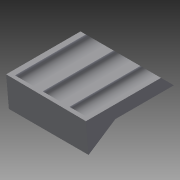
# Autodesk Inventor part: coin_holder_large_only
Saved by Autodesk Inventor 2015 (Build 190159000, 159)
## iProperties
Created: 2015-02-10
Part Number: coin_holder_large_only
Material: Generic
Document SubType Name: Modeling
Designer: Justin
Density: 1 g/cm^3
Appearance: Default
Author: Justin
Autodesk Inventor part; units mm, degrees
ref_plane "YZ Plane" through (0, 0, 0) normal (1, 0, 0) x (0, 1, 0)
ref_plane "XZ Plane" through (0, 0, 0) normal (0, 1, 0) x (-1, 0, 0)
sketch "Sketch1" plane through (0, 0, 0) normal (0, 0, 1) x (1, 0, 0)
  arc A0 (12.7973, -6.8176) -> (-12.597, -7.1809) centre (0, 0) ccw
  arc A1 (50.4829, -6.2785) -> (26.2017, -6.6259) centre (38.25, 0) ccw
  arc A2 (85.5853, -5.7763) -> (63.5844, -6.091) centre (74.5, 0) ccw
  arc A3 (117.8988, -5.314) -> (98.5072, -5.5914) centre (108.125, 0) ccw
  arc A4 (147.9764, -4.8837) -> (130.6669, -5.1313) centre (139.25, 0) ccw
  arc A5 (177.1345, -4.4665) -> (160.4967, -4.7045) centre (168.75, 0) ccw
  line L0 (-20, 20) -> (188.75, 20)
  line L1 (188.75, 20) -> (188.75, -4.3003)
  line L2 (-20, 20) -> (-20, -7.2868)
  line L3 (-20, -7.2868) -> (188.75, -4.3003)
  dimension "d0" = 29
  dimension "d1" = 27.5
  dimension "d2" = 25
  dimension "d3" = 22.25
  dimension "d4" = 20
  dimension "d5" = 19
  dimension "d6" = 38.25
  dimension "d7" = 36.25
  dimension "d8" = 33.625
  dimension "d9" = 31.125
  dimension "d10" = 29.5
  dimension "d11" = 0
  dimension "d12" = 0
  dimension "d13" = 0
  dimension "d14" = 0
  dimension "d15" = 0
  dimension "d20" = 20
  dimension "d22" = 20
  dimension "d23" = 20
  dimension "d24" = 7
  dimension "d25" = 4.586
  constraints: 12 point on circle, 6 centre point, 6 end point, 1 coincident, 1 horizontal, 1 perpendicular, 1 vertical, 15 other
  measures "d0" diameter of A0
  measures "d1" diameter of A1
  measures "d2" diameter of A2
  measures "d3" diameter of A3
  measures "d4" diameter of A4
  measures "d5" diameter of A5
  measures "d6" distance of A1.centre A0.centre
  measures "d7" distance of A2.centre A1.centre
  measures "d8" distance of A3.centre A2.centre
  measures "d9" distance of A4.centre A3.centre
  measures "d10" distance of A5.centre A4.centre
  measures "d11" vertical distance of point (0, 0) A1.centre
  measures "d12" vertical distance of A1.centre A2.centre
  measures "d13" vertical distance of A2.centre A3.centre
  measures "d14" vertical distance of A3.centre A4.centre
  measures "d15" vertical distance of A4.centre A5.centre
  measures "d20" distance from line of L0 A0.centre
  measures "d22" horizontal distance of A5.centre L0.end
  measures "d23" distance from line of L2 A0.centre
sketch "Sketch4" plane through (0, 0, 0) normal (1, 0, 0) x (0, 1, 0)
  line L0 (0, 0) -> (29.9033, -29.9033)
  line L1 (0, 5.9807) -> (0, -35.884) projected
  point P0 (100, 0)
  dimension "d51" = 45
  dimension "d53" = 0
  dimension "d55" = 29.9033
  dimension "d98" = 100
  constraints: 2 end point
  measures "d51" angle of L0 L1
  measures "d53" vertical distance of L0.start point (100, 0)
  measures "d55" horizontal distance of L0.start L0.end
  measures "d98" distance of L0.start point (100, 0)
ref_plane "Work Plane4" through (0, 100, 0) normal (0, 0.7071068, 0.7071068) x (1, 0, 0)
ref_plane "Work Plane3" through (-10, 0, 0) normal (0, 0.7071068, 0.7071068) x (1, 0, 0)
sketch "Sketch5" plane through (-10, 0, 0) normal (0, 0.7071068, 0.7071068) x (1, 0, 0)
  arc A0 (42.7973, 0.4692) -> (17.403, 0.1059) centre (30, 7.2868) ccw
  arc A1 (80.4829, 1.0084) -> (56.2017, 0.661) centre (68.25, 7.2868) ccw
  arc A2 (115.5853, 1.5106) -> (93.5844, 1.1958) centre (104.5, 7.2868) ccw
  arc A3 (147.8988, 1.9729) -> (128.5072, 1.6954) centre (138.125, 7.2868) ccw
  arc A4 (177.9764, 2.4032) -> (160.6669, 2.1555) centre (169.25, 7.2868) ccw
  arc A5 (207.1345, 2.8203) -> (190.4967, 2.5823) centre (198.75, 7.2868) ccw
  line L0 (10, 27.2868) -> (218.75, 27.2868)
  line L1 (218.75, 27.2868) -> (218.75, 2.9865)
  line L2 (10, 27.2868) -> (10, 0)
  line L3 (10, 0) -> (17.403, 0.1059)
  line L4 (42.7973, 0.4692) -> (56.2017, 0.661)
  line L5 (80.4829, 1.0084) -> (93.5844, 1.1958)
  line L6 (115.5853, 1.5106) -> (128.5072, 1.6954)
  line L7 (207.1345, 2.8203) -> (218.75, 2.9865)
  line L8 (147.8988, 1.9729) -> (160.6669, 2.1555)
  line L9 (177.9764, 2.4032) -> (190.4967, 2.5823)
  dimension "d56" = 29
  dimension "d57" = 27.5
  dimension "d58" = 25
  dimension "d59" = 22.25
  dimension "d60" = 20
  dimension "d61" = 19
  dimension "d62" = 38.25
  dimension "d63" = 36.25
  dimension "d64" = 33.625
  dimension "d65" = 31.125
  dimension "d66" = 29.5
  dimension "d67" = 0
  dimension "d68" = 0
  dimension "d69" = 0
  dimension "d70" = 0
  dimension "d71" = 0
  dimension "d72" = 20
  dimension "d73" = 20
  dimension "d74" = 20
  constraints: 20 end point, 12 point on circle, 6 centre point, 2 coincident, 1 horizontal, 1 perpendicular, 1 vertical
  measures "d56" diameter of A0
  measures "d57" diameter of A1
  measures "d58" diameter of A2
  measures "d59" diameter of A3
  measures "d60" diameter of A4
  measures "d61" diameter of A5
  measures "d62" distance of A1.centre A0.centre
  measures "d63" distance of A2.centre A1.centre
  measures "d64" distance of A3.centre A2.centre
  measures "d65" distance of A4.centre A3.centre
  measures "d66" distance of A5.centre A4.centre
  measures "d67" vertical distance of point (30, 7.287) A1.centre
  measures "d68" vertical distance of A1.centre A2.centre
  measures "d69" vertical distance of A2.centre A3.centre
  measures "d70" vertical distance of A3.centre A4.centre
  measures "d71" vertical distance of A4.centre A5.centre
  measures "d72" distance from line of L0 A0.centre
  measures "d73" horizontal distance of A5.centre L0.end
  measures "d74" distance from line of L2 A0.centre
sketch "Sketch6" plane through (0, 100, 0) normal (0, 0.7071068, 0.7071068) x (1, 0, 0)
  arc A0 (32.7973, 0.4692) -> (7.403, 0.1059) centre (20, 7.2868) ccw
  arc A1 (70.4829, 1.0084) -> (46.2017, 0.661) centre (58.25, 7.2868) ccw
  arc A2 (105.5853, 1.5106) -> (83.5844, 1.1958) centre (94.5, 7.2868) ccw
  arc A3 (137.8988, 1.9729) -> (118.5072, 1.6954) centre (128.125, 7.2868) ccw
  arc A4 (167.9764, 2.4032) -> (150.6669, 2.1555) centre (159.25, 7.2868) ccw
  arc A5 (197.1345, 2.8203) -> (180.4967, 2.5823) centre (188.75, 7.2868) ccw
  line L0 (0, 27.2868) -> (208.75, 27.2868)
  line L1 (208.75, 27.2868) -> (208.75, 2.9865)
  line L2 (0, 27.2868) -> (0, 0)
  line L3 (0, 0) -> (7.403, 0.1059)
  line L4 (32.7973, 0.4692) -> (46.2017, 0.661)
  line L5 (70.4829, 1.0084) -> (83.5844, 1.1958)
  line L6 (105.5853, 1.5106) -> (118.5072, 1.6954)
  line L7 (137.8988, 1.9729) -> (150.6669, 2.1555)
  line L8 (167.9764, 2.4032) -> (180.4967, 2.5823)
  line L9 (197.1345, 2.8203) -> (208.75, 2.9865)
  point P0 (0, -70.7107)
  dimension "d77" = 29
  dimension "d78" = 27.5
  dimension "d79" = 25
  dimension "d80" = 22.25
  dimension "d81" = 20
  dimension "d82" = 19
  dimension "d83" = 38.25
  dimension "d84" = 36.25
  dimension "d85" = 33.625
  dimension "d86" = 31.125
  dimension "d87" = 29.5
  dimension "d88" = 0
  dimension "d89" = 0
  dimension "d90" = 0
  dimension "d91" = 0
  dimension "d92" = 0
  dimension "d93" = 20
  dimension "d94" = 20
  dimension "d95" = 20
  constraints: 20 end point, 12 point on circle, 6 centre point, 2 coincident, 1 horizontal, 1 perpendicular, 1 vertical
  measures "d77" diameter of A0
  measures "d78" diameter of A1
  measures "d79" diameter of A2
  measures "d80" diameter of A3
  measures "d81" diameter of A4
  measures "d82" diameter of A5
  measures "d83" distance of A1.centre A0.centre
  measures "d84" distance of A2.centre A1.centre
  measures "d85" distance of A3.centre A2.centre
  measures "d86" distance of A4.centre A3.centre
  measures "d87" distance of A5.centre A4.centre
  measures "d88" vertical distance of point (20, 7.287) A1.centre
  measures "d89" vertical distance of A1.centre A2.centre
  measures "d90" vertical distance of A2.centre A3.centre
  measures "d91" vertical distance of A3.centre A4.centre
  measures "d92" vertical distance of A4.centre A5.centre
  measures "d93" distance from line of L0 A0.centre
  measures "d94" horizontal distance of A5.centre L0.end
  measures "d95" distance from line of L2 A0.centre
loft "Loft1" add profiles "Sketch6", "Sketch5"
sketch "Sketch7" plane through (0, 0, 0) normal (0, 1, 0) x (-1, 0, 0)
  line L0 (0, 0) -> (0, -19.2947) projected
  line L1 (0, -19.2947) -> (-208.75, -19.2947) projected
  line L2 (-208.75, -19.2947) -> (-208.75, -2.1118) projected
  line L3 (-208.75, -2.1118) -> (-197.1345, -1.9943) projected
  ellipse E0 centre (-188.75, -5.1526) end of major axis (-198.25, -5.1526) minor radius 6.7175 (-197.1345, -1.9943) -> (-180.4967, -1.826) ccw projected
  line L4 (-180.4967, -1.826) -> (-167.9764, -1.6993) projected
  ellipse E1 centre (-159.25, -5.1526) end of major axis (-169.25, -5.1526) minor radius 7.0711 (-167.9764, -1.6993) -> (-150.6669, -1.5242) ccw projected
  line L5 (-150.6669, -1.5242) -> (-137.8988, -1.395) projected
  ellipse E2 centre (-128.125, -5.1526) end of major axis (-139.25, -5.1526) minor radius 7.8666 (-137.8988, -1.395) -> (-118.5072, -1.1989) ccw projected
  line L6 (-118.5072, -1.1989) -> (-105.5853, -1.0681) projected
  ellipse E3 centre (-94.5, -5.1526) end of major axis (-107, -5.1526) minor radius 8.8388 (-105.5853, -1.0681) -> (-83.5844, -0.8456) ccw projected
  line L7 (-83.5844, -0.8456) -> (-70.4829, -0.713) projected
  ellipse E4 centre (-58.25, -5.1526) end of major axis (-72, -5.1526) minor radius 9.7227 (-70.4829, -0.713) -> (-46.2017, -0.4674) ccw projected
  line L8 (-46.2017, -0.4674) -> (-32.7973, -0.3318) projected
  ellipse E5 centre (-20, -5.1526) end of major axis (-34.5, -5.1526) minor radius 10.253 (-32.7973, -0.3318) -> (-7.403, -0.0749) ccw projected
  line L9 (-7.403, -0.0749) -> (0, 0) projected
  line L10 (0, 0) -> (0, -19.2947)
  line L11 (0, -19.2947) -> (-208.75, -19.2947)
  line L12 (-208.75, -19.2947) -> (-208.75, -2.1118)
  line L13 (-208.75, -2.1118) -> (0, 0)
  constraints: 8 end point, 1 collinear, 1 perpendicular, 1 vertical, 6 other
sketch "Sketch10" plane through (0, 19.2947, -19.2947) normal (-1, 0, 0) x (0, 0, 1)
  line L0 (19.2947, 80.7053) -> (0, 100) projected
  line L1 (0, 100) -> (0, 0) projected
  line L2 (19.2947, -19.2947) -> (0, 0) projected
  line L3 (19.2947, 80.7053) -> (19.2947, -19.2947) projected
  line L4 (19.2947, -19.2947) -> (19.2947, -24.2947)
  line L5 (0, 0) -> (0, -22.6066)
  line L6 (0, -22.6066) -> (19.2947, -24.2947)
  line L7 (0, -22.6066) -> (-24.9049, -20.4278)
  line L8 (-24.9049, -20.4278) -> (0, 17.5461)
  line L9 (0, 100) -> (0, 0) projected
  line L10 (0, 17.5461) -> (0, 0)
  point P0 (19.2947, -19.2947)
  dimension "d106" = 5
  dimension "d111" = 85
  dimension "d113" = 25
  dimension "d114" = 40
  constraints: 12 end point, 3 vertical, 1 collinear, 1 point on line
  measures "d106" distance of L2.start L4.end
  measures "d111" angle of L5 L6
  measures "d113" distance of L5.end L7.end
  measures "d114" distance from line of L7 L8.end
sketch "Sketch11" plane through (208.75, 2.1118, -2.1118) normal (1, 0, 0) x (0, 0, -1)
  line L0 (17.1829, 117.1829) -> (0, 100) projected
  line L1 (0, 100) -> (0, 0) projected
  line L2 (17.1829, 17.1829) -> (0, 0) projected
  line L3 (17.1829, 117.1829) -> (17.1829, 17.1829) projected
  line L4 (17.1829, 17.1829) -> (0, 0)
  line L5 (10.1119, 10.1119) -> (-0.5876, -0.5876) projected
  line L6 (17.1829, -5.4237) -> (-2.1118, -7.1118) projected
  line L7 (0, 0) -> (0, -6.927)
  line L8 (17.1829, -5.4237) -> (0, -6.927)
  line L9 (17.1829, -5.4237) -> (17.1829, 17.1829)
  line L10 (0, -6.927) -> (17.1829, -5.4237)
  line L11 (17.1829, -5.4237) -> (42.0878, -3.2448)
  line L12 (42.0878, -3.2448) -> (17.1829, 34.5763)
  line L13 (17.1829, 117.1829) -> (17.1829, 17.1829) projected
  line L14 (17.1829, 17.1829) -> (17.1829, 34.5763)
  point P0 (-2.1118, -2.1118)
  point P1 (17.1829, -7.1118)
  point P2 (-0.4125, -0.4125)
  dimension "d115" = 25
  dimension "d116" = 40
  constraints: 16 end point, 5 collinear, 2 point on line, 2 vertical
  measures "d115" distance of L8.start L11.end
  measures "d116" distance of L6.start L12.end
loft "Loft3" add profiles "Sketch10", "Sketch11" contours L4 L6 L5 L2 | L1 L5 L7 L8 / L12 L11 L9 L3 | L2 L9 L6 L7
sketch "Sketch13" plane through (0, -1.133, -44.1996) normal (0, -0.9961947, -0.0871557) x (1, 0, 0)
  line L0 (0, 35.2171) -> (0, 14.3141) projected
  line L1 (7.403, 35.1359) -> (0, 35.2171) projected
  ellipse E0 centre (20, 29.635) end of major axis (5.5, 29.635) minor radius 11.1076 (7.403, 35.1359) -> (32.7973, 34.8576) ccw projected
  line L2 (46.2017, 34.7107) -> (32.7973, 34.8576) projected
  ellipse E1 centre (58.25, 29.635) end of major axis (44.5, 29.635) minor radius 10.5331 (46.2017, 34.7107) -> (70.4829, 34.4446) ccw projected
  line L3 (83.5844, 34.301) -> (70.4829, 34.4446) projected
  ellipse E2 centre (94.5, 29.635) end of major axis (82, 29.635) minor radius 9.5756 (83.5844, 34.301) -> (105.5853, 34.0599) ccw projected
  line L4 (118.5072, 33.9183) -> (105.5853, 34.0599) projected
  ellipse E3 centre (128.125, 29.635) end of major axis (117, 29.635) minor radius 8.5222 (118.5072, 33.9183) -> (137.8988, 33.7058) ccw projected
  line L5 (150.6669, 33.5658) -> (137.8988, 33.7058) projected
  ellipse E4 centre (159.25, 29.635) end of major axis (149.25, 29.635) minor radius 7.6604 (150.6669, 33.5658) -> (167.9764, 33.3761) ccw projected
  line L6 (180.4967, 33.2389) -> (167.9764, 33.3761) projected
  ellipse E5 centre (188.75, 29.635) end of major axis (179.25, 29.635) minor radius 7.2774 (180.4967, 33.2389) -> (197.1345, 33.0566) ccw projected
  line L7 (208.75, 32.9293) -> (197.1345, 33.0566) projected
  line L8 (208.75, 14.3141) -> (208.75, 32.9293) projected
  line L9 (0, 14.3141) -> (208.75, 14.3141) projected
  line L10 (0, 0) -> (0, 44.3684) projected
  line L11 (0, 0) -> (208.75, 0) projected
  line L12 (208.75, 0) -> (208.75, 42.2486) projected
  line L13 (0, 44.3684) -> (208.75, 42.2486) projected
  line L14 (0, 0) -> (208.75, 0) projected
  line L15 (112.5, 0) -> (112.5, 43.226)
  point P0 (0, 43.9326)
  dimension "d122" = 18
  constraints: 2 end point, 2 point on line, 1 perpendicular, 6 other
  measures "d122" distance from line of point (94.5, 29.635) L15
split body "Split1" sketch "Sketch13" result one side removed curves L15 removed pieces at (176.6667, 64.2471, -18.7947)
body "Solid2"
